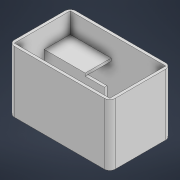
# Autodesk Inventor part: Bike_Telemetry
Saved by Autodesk Inventor 2022 (Build 260153000, 153)
## iProperties
Created: 2022-06-22
Part Number: Bike_Telemetry
Material: Generic
Document SubType Name: Modeling
Designer: Gugarauj07
Density: 1 g/cm^3
Appearance: Default
Author: Gugarauj07
Autodesk Inventor part; units mm, degrees
ref_plane "YZ Plane" through (0, 0, 0) normal (1, 0, 0) x (0, 1, 0)
ref_plane "XZ Plane" through (0, 0, 0) normal (0, 1, 0) x (-1, 0, 0)
ref_plane "XY Plane" through (0, 0, 0) normal (0, 0, 1) x (1, 0, 0)
sketch "Sketch1" plane through (0, 0, 0) normal (0, 0, 1) x (1, 0, 0)
  line L0 (0, 0) -> (74, 0)
  line L1 (74, 0) -> (74, 45)
  line L2 (74, 45) -> (0, 45)
  line L3 (0, 45) -> (0, 0)
  dimension "d3" = 74
  dimension "d4" = 45
  constraints: 8 end point, 2 parallel, 1 horizontal, 1 perpendicular, 1 vertical
  measures "d3" distance of L2.end L1.end
  measures "d4" distance of L1.end L0.end
extrude "Extrusion1" add sketch "Sketch1" along normal blind 45
shell "Shell1" thickness 2 removed faces 1 at (49.3333, 45, 30)
sketch "Sketch2" plane through (2, 2, 2) normal (0, 1, 0) x (1, 0, 0)
  line L0 (70, -41) -> (0, -41) projected
  line L1 (0, -41) -> (10, -41)
  line L2 (10, -41) -> (42, -41)
  line L3 (42, -41) -> (42, -31)
  line L4 (42, -31) -> (10, -31)
  line L5 (10, -31) -> (10, -41)
  line L6 (70, 0) -> (70, -41) projected
  line L7 (0, -41) -> (0, 0) projected
  point P0 (-2, 2)
  dimension "d9" = 32
  dimension "d10" = 10
  dimension "d11" = 70
  constraints: 10 end point, 2 parallel, 1 horizontal, 1 perpendicular, 1 point on line
  measures "d9" distance of L4.end L3.end
  measures "d10" distance of L3.end L2.end
  measures "d11" distance between parallel lines of L6 L7
extrude "Extrusion2" cut sketch "Sketch2" against normal through all
sketch "Sketch3" plane through (2, 2, 2) normal (0, 1, 0) x (1, 0, 0)
  line L0 (0, 0) -> (0, -41) projected
  line L1 (0, -17) -> (0, 33)
  line L2 (0, -17) -> (44, -17)
  line L3 (44, -17) -> (0, -17)
  line L4 (0, -17) -> (0, -19)
  line L5 (0, -19) -> (44, -19)
  line L6 (44, -19) -> (44, -17)
  point P0 (-2, 2)
  dimension "d16" = 44
  dimension "d17" = 2
  constraints: 12 end point, 2 horizontal, 2 parallel, 2 point on line, 1 collinear, 1 perpendicular
  measures "d16" distance of L1.start L2.end
  measures "d17" distance of L4.end L3.end
extrude "Extrusion3" add sketch "Sketch3" along normal blind 26
fillet "Fillet1" radius 4 1 edges at (0, 22.5, 0)
fillet "Fillet2" radius 4 1 edges at (74, 22.5, 0)
fillet "Fillet3" radius 4 1 edges at (74, 22.5, 45)
fillet "Fillet4" radius 4 1 edges at (0, 22.5, 45)
sketch "Sketch4" plane through (2, 2, 2) normal (1, 0, 0) x (0, 0, -1)
  line L0 (-19, 26) -> (-17, 26) projected
  line L1 (-19, 26) -> (0, 26)
  line L2 (0, 26) -> (0, 28)
  line L3 (0, 28) -> (-19, 28)
  line L4 (-19, 28) -> (-19, 26)
  point P0 (2, -2)
  dimension "d24" = 2
  constraints: 8 end point, 2 parallel, 1 horizontal, 1 perpendicular
  measures "d24" distance of L2.end L1.end
extrude "Extrusion4" add sketch "Sketch4" along normal blind 30
sketch "Sketch6" plane through (2, 2, 2) normal (0, 0, 1) x (1, 0, 0)
  point P0 (-2, -2)
body "Solid1"
